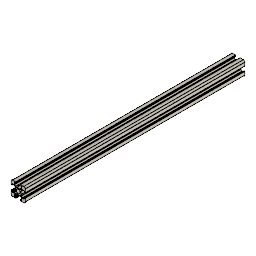
2020_Extrusion_Bed_sides_F01 (Autodesk Fusion 360 design; units mm, degrees)
Autodesk Fusion 360 part; units mm, degrees
sketch "スケッチ1" plane through (0, 0, 0) normal (0, 1, 0) x (1, 0, 0)
  line L0 (8, 10) -> (-8, 10)
  line L1 (-10, 8) -> (-10, -8)
  line L2 (-8, -10) -> (8, -10)
  line L3 (10, -8) -> (10, 8)
  line L4 (10, 10) -> (-10, -10) construction
  line L5 (-10, 10) -> (10, -10) construction
  circle A0 centre (0, 0) radius 2.6
  line L6 (-3.2, -10) -> (-3.2, -8.65)
  line L7 (-3.2, -8.65) -> (-4.6, -8.65)
  line L8 (-5.1, -8.15) -> (-5.1, -6.3678)
  line L9 (-4.9536, -6.0142) -> (-3.4251, -4.4858)
  line L10 (0, 0) -> (0, -10) construction
  line L11 (-2.0109, -3.9) -> (0, -3.9)
  arc A1 (-5.1, -8.15) -> (-4.6, -8.65) centre (-4.6, -8.15) ccw
  arc A2 (-4.9536, -6.0142) -> (-5.1, -6.3678) centre (-4.6, -6.3678) ccw
  arc A3 (-2.0109, -3.9) -> (-3.4251, -4.4858) centre (-2.0109, -5.9) ccw
  arc A4 (-10, -8) -> (-8, -10) centre (-8, -8) ccw
  arc A5 (10, 8) -> (8, 10) centre (8, 8) ccw
  arc A6 (8, -10) -> (10, -8) centre (8, -8) ccw
  arc A7 (-8, 10) -> (-10, 8) centre (-8, 8) ccw
  line L12 (3.2, -10) -> (3.2, -8.65)
  line L13 (3.2, -8.65) -> (4.6, -8.65)
  arc A8 (4.6, -8.65) -> (5.1, -8.15) centre (4.6, -8.15) ccw
  line L14 (5.1, -8.15) -> (5.1, -6.3678)
  arc A9 (5.1, -6.3678) -> (4.9536, -6.0142) centre (4.6, -6.3678) ccw
  line L15 (4.9536, -6.0142) -> (3.4251, -4.4858)
  arc A10 (3.4251, -4.4858) -> (2.0109, -3.9) centre (2.0109, -5.9) ccw
  line L16 (2.0109, -3.9) -> (0, -3.9)
  line L17 (10, -3.2) -> (8.65, -3.2)
  line L18 (8.65, -3.2) -> (8.65, -4.6)
  arc A11 (8.15, -5.1) -> (8.65, -4.6) centre (8.15, -4.6) ccw
  line L19 (8.15, -5.1) -> (6.3678, -5.1)
  arc A12 (6.0142, -4.9536) -> (6.3678, -5.1) centre (6.3678, -4.6) ccw
  line L20 (6.0142, -4.9536) -> (4.4858, -3.4251)
  arc A13 (3.9, -2.0109) -> (4.4858, -3.4251) centre (5.9, -2.0109) ccw
  line L21 (3.9, -2.0109) -> (3.9, 0)
  line L22 (3.9, 2.0109) -> (3.9, 0)
  arc A14 (4.4858, 3.4251) -> (3.9, 2.0109) centre (5.9, 2.0109) ccw
  line L23 (6.0142, 4.9536) -> (4.4858, 3.4251)
  arc A15 (6.3678, 5.1) -> (6.0142, 4.9536) centre (6.3678, 4.6) ccw
  line L24 (8.15, 5.1) -> (6.3678, 5.1)
  arc A16 (8.65, 4.6) -> (8.15, 5.1) centre (8.15, 4.6) ccw
  line L25 (8.65, 3.2) -> (8.65, 4.6)
  line L26 (10, 3.2) -> (8.65, 3.2)
  line L27 (3.2, 10) -> (3.2, 8.65)
  line L28 (3.2, 8.65) -> (4.6, 8.65)
  arc A17 (5.1, 8.15) -> (4.6, 8.65) centre (4.6, 8.15) ccw
  line L29 (5.1, 8.15) -> (5.1, 6.3678)
  arc A18 (4.9536, 6.0142) -> (5.1, 6.3678) centre (4.6, 6.3678) ccw
  line L30 (4.9536, 6.0142) -> (3.4251, 4.4858)
  arc A19 (2.0109, 3.9) -> (3.4251, 4.4858) centre (2.0109, 5.9) ccw
  line L31 (2.0109, 3.9) -> (0, 3.9)
  line L32 (-2.0109, 3.9) -> (0, 3.9)
  arc A20 (-3.4251, 4.4858) -> (-2.0109, 3.9) centre (-2.0109, 5.9) ccw
  line L33 (-4.9536, 6.0142) -> (-3.4251, 4.4858)
  arc A21 (-5.1, 6.3678) -> (-4.9536, 6.0142) centre (-4.6, 6.3678) ccw
  line L34 (-5.1, 8.15) -> (-5.1, 6.3678)
  arc A22 (-4.6, 8.65) -> (-5.1, 8.15) centre (-4.6, 8.15) ccw
  line L35 (-3.2, 8.65) -> (-4.6, 8.65)
  line L36 (-3.2, 10) -> (-3.2, 8.65)
  line L37 (-10, 3.2) -> (-8.65, 3.2)
  line L38 (-8.65, 3.2) -> (-8.65, 4.6)
  arc A23 (-8.15, 5.1) -> (-8.65, 4.6) centre (-8.15, 4.6) ccw
  line L39 (-8.15, 5.1) -> (-6.3678, 5.1)
  arc A24 (-6.0142, 4.9536) -> (-6.3678, 5.1) centre (-6.3678, 4.6) ccw
  line L40 (-6.0142, 4.9536) -> (-4.4858, 3.4251)
  arc A25 (-3.9, 2.0109) -> (-4.4858, 3.4251) centre (-5.9, 2.0109) ccw
  line L41 (-3.9, 2.0109) -> (-3.9, 0)
  line L42 (-3.9, -2.0109) -> (-3.9, 0)
  arc A26 (-4.4858, -3.4251) -> (-3.9, -2.0109) centre (-5.9, -2.0109) ccw
  line L43 (-6.0142, -4.9536) -> (-4.4858, -3.4251)
  arc A27 (-6.3678, -5.1) -> (-6.0142, -4.9536) centre (-6.3678, -4.6) ccw
  line L44 (-8.15, -5.1) -> (-6.3678, -5.1)
  arc A28 (-8.65, -4.6) -> (-8.15, -5.1) centre (-8.15, -4.6) ccw
  line L45 (-8.65, -3.2) -> (-8.65, -4.6)
  line L46 (-10, -3.2) -> (-8.65, -3.2)
  dimension "d1" = 20
  dimension "d2" = 20
  dimension "d3" = 5.2
  dimension "d4" = 1.35
  dimension "d5" = 3.2
  dimension "d6" = 5.1
  dimension "d7" = 6.1
  dimension "d8" = 0.75
  dimension "d9" = 0.5
  dimension "d10" = 2
  dimension "d11" = 2
  dimension "d12" = 2
  dimension "d13" = 2
  dimension "d14" = 2
  dimension "d16" = 360
  measures "d3" diameter of A0
  measures "d5" distance of L6 L10
  measures "d6" distance of L8 L10
  measures "d7" distance of L2 L11
  measures "d8" distance of L4 L9
  measures "d9" radius of A1
  measures "d10" radius of A3
  measures "d11" radius of A4
  measures "d12" radius of A5
  measures "d13" radius of A6
  measures "d14" radius of A7
extrude "押し出し1" add sketch "スケッチ1" along normal mid plane 310 contours L0 L1 L2 L3 L6 L7 L8 L9 L11 A1 A2 A3 A4 A5 A6 A7 L12 L13 A8 L14 A9 L15 A10 L16 L17 L18 A11 L19 A12 L20 A13 L21 L22 A14 L23 A15 L24 A16 L25 L26 L27 L28 A17 L29 A18 L30 A19 L31 L32 A20 L33 A21 L34 A22 L35 L36 L37 L38 A23 L39 A24 L40 A25 L41 L42 A26 L43 A27 L44 A28 L45 L46
